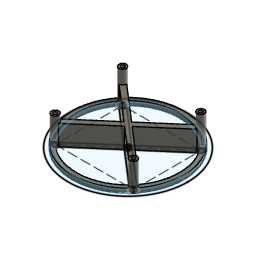
Sat Stand 2 (Autodesk Fusion 360 design; units mm, degrees)
Autodesk Fusion 360 part; units mm, degrees
note: some values were not read from the file. Set by a fixed rule: which sketch regions a step uses.
sketch "Sketch1" plane through (0, 0, 0) normal (0, 1, 0) x (1, 0, 0)
  circle A0 centre (0, 0) radius 44
  line L0 (28.875, 24.875) -> (-28.875, 24.875) construction
  line L1 (-28.875, 24.875) -> (-28.875, -24.875) construction
  line L2 (-28.875, -24.875) -> (28.875, -24.875) construction
  line L3 (28.875, -24.875) -> (28.875, 24.875) construction
  line L4 (28.875, 24.875) -> (-28.875, -24.875) construction
  line L5 (-28.875, 24.875) -> (28.875, -24.875) construction
  circle A1 centre (-28.875, 24.875) radius 1.375
  circle A2 centre (-28.875, 24.875) radius 2.75
  circle A3 centre (-28.875, -24.875) radius 1.375
  circle A4 centre (-28.875, -24.875) radius 2.75
  circle A5 centre (28.875, 24.875) radius 1.375
  circle A6 centre (28.875, 24.875) radius 2.75
  circle A7 centre (28.875, -24.875) radius 1.375
  circle A8 centre (28.875, -24.875) radius 2.75
  line L6 (-30.4443, 23.5871) -> (27.8036, -26.5919)
  line L7 (-27.8037, 26.5919) -> (30.4442, -23.5871)
  line L8 (27.8041, 26.5923) -> (-30.4447, -23.5875)
  line L9 (30.4447, 23.5875) -> (-27.8041, -26.5923)
  circle A9 centre (0, 0) radius 40.9963
  circle A10 centre (0, 0) radius 37.9963
  dimension "d1" = 88
  dimension "d2" = 57.75
  dimension "d3" = 49.75
  dimension "d4" = 2.75
  dimension "d5" = 5.5
  dimension "d6" = 2.75
  dimension "d7" = 5.5
  dimension "d8" = 2.75
  dimension "d9" = 5.5
  dimension "d10" = 2.75
  dimension "d11" = 5.5
  dimension "d26" = 2
  dimension "d27" = -2
  dimension "d28" = 2
  dimension "d29" = -2
  dimension "d30" = -3
  constraint coincident A0.centre A9.centre
  constraint horizontal L0
  constraint perpendicular L0 L1
  constraint parallel L0 L2
  constraint parallel L1 L3
  constraint coincident L4 A0.centre
  constraint coincident L5 A0.centre
  constraint coincident L0.end L1.start
  constraint concentric A1 A2
  constraint coincident L1.end L2.start
  constraint concentric A3 A4
  constraint coincident L0.start L3.end
  constraint concentric A5 A6
  constraint coincident L2.end L3.start
  constraint concentric A7 A8
  constraint concentric A0 A9
  measures "d1" diameter of A0
  measures "d2" distance of L1.end L2.end
  measures "d3" distance of L0.end L1.end
  measures "d4" diameter of A1
  measures "d5" diameter of A2
  measures "d6" diameter of A3
  measures "d7" diameter of A4
  measures "d8" diameter of A5
  measures "d9" diameter of A6
  measures "d10" diameter of A7
  measures "d11" diameter of A8
extrude "Extrude7" add sketch "Sketch1" along normal blind 3 contours A9 makes body 1
extrude "Extrude8" add sketch "Sketch1" along normal blind 15 separate body contours A1 A10 | A1 A10 | A2 L6 L7 L8 | A6 L7 L8 L9 | L6 L7 L8 L9 | A4 L6 L8 L9 | A8 L6 L7 L9 | A5 A10 | A5 A10 | A3 A10 | A3 A10 | A7 A10 | A7 A10 makes body 2 at (-27.5068, 10, -25.0119) makes body 3 at (30.2432, 5, -24.7381) makes body 4 at (-29.6776, 10, 25.9914) makes body 5 at (9.9096, 0, 8.6263) makes body 6 at (30.2432, 5, 25.0119)
extrude "Extrude9" add sketch "Sketch1" along normal blind 20 contours A3 A4 A10 | A4 L8 A10 | A3 A4 L8 L9 A10 | A4 L9 A10 | A7 A8 L6 L7 A10 | A8 L7 A10 | A8 L6 A10 | A7 A8 A10 bodies 1 4 5 6
extrude "Extrude10" add sketch "Sketch1" along normal blind 25 contours A1 A2 L6 L7 A10 | A1 A2 A10 | A2 L7 A10 | A2 L6 A10 | A6 L8 A10 | A5 A6 A10 | A5 A6 L8 L9 A10 | A6 L9 A10 bodies 1 2 3
equation "d2 = 55 mm + 2.75 mm"
equation "d3 = 48 mm + 1.75 mm"
named bodies: "sat stand 2"
